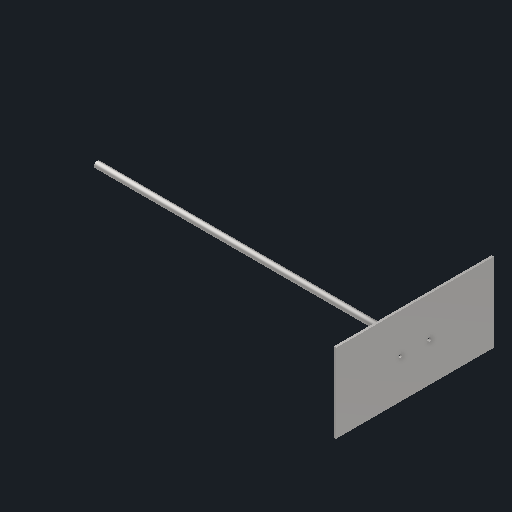
# Autodesk Inventor part: Screw
Saved by Autodesk Inventor 2023 (Build 270158000, 158)
## iProperties
Created: 2023-11-09
Part Number: Screw
Material: Generic
Document SubType Name: Modeling
Designer: Abhinav
Density: 1 g/cm^3
Appearance: Stainless - Brushed
Author: Abhinav
Autodesk Inventor part; units mm, degrees
ref_plane "YZ Plane" through (0, 0, 0) normal (1, 0, 0) x (0, 1, 0)
ref_plane "XZ Plane" through (0, 0, 0) normal (0, 1, 0) x (-1, 0, 0)
ref_plane "XY Plane" through (0, 0, 0) normal (0, 0, 1) x (1, 0, 0)
sketch "Sketch1" plane through (0, 0, 0) normal (1, 0, 0) x (0, 1, 0)
  circle A0 centre (0, 0) radius 4
  dimension "d0" = 8
  constraints: 1 centre point, 1 coincident
  measures "d0" diameter of A0
extrude "Extrusion1" add sketch "Sketch1" along normal blind 400
sketch "Sketch2" plane through (400, 0, 0) normal (1, 0, 0) x (0, 0, -1)
  line L0 (-100, 50) -> (100, 50)
  line L1 (100, 50) -> (100, -50)
  line L2 (100, -50) -> (-100, -50)
  line L3 (-100, -50) -> (-100, 50)
  circle A0 centre (0, 0) radius 4 projected
  line L4 (-100, 50) -> (100, -50) construction
  line L5 (100, 50) -> (-100, -50) construction
  line L6 (0, 0) -> (-18.25, 0) construction
  circle A1 centre (-18.25, 0) radius 2.6
  circle A2 centre (0, 0) radius 4 construction
  line L7 (0, 0) -> (18.25, 0) construction
  circle A3 centre (18.25, 0) radius 2.6
  dimension "d3" = 200
  dimension "d4" = 100
  dimension "d7" = 18.25
  dimension "d8" = 5.2
  constraints: 16 end point, 3 horizontal, 2 centre point, 2 coincident, 2 midpoint, 2 parallel, 1 collinear, 1 equal radius, 1 perpendicular
  measures "d3" distance of L1.end L2.end
  measures "d4" distance of L0.end L1.end
  measures "d7" distance of L6.start L6.end
  measures "d8" diameter of A1
extrude "Extrusion2" add sketch "Sketch2" along normal blind 3 contours L0 L1 L2 L3 | A0
body "Solid1"
